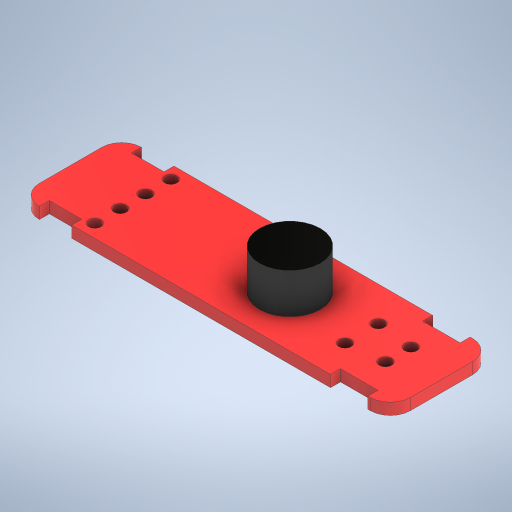
# Autodesk Inventor part: femtobuck-sparkfun
Saved by Autodesk Inventor 2023 (Build 270158030, 158C)
## iProperties
Created: 2023-08-09
Part Number: femtobuck-sparkfun
Material: Generic
Document SubType Name: Modeling
Designer: Imogen Heard
Density: 1 g/cm^3
Appearance: Default
Author: Imogen Heard
Autodesk Inventor part; units mm, degrees
ref_plane "YZ Plane" through (0, 0, 0) normal (1, 0, 0) x (0, 1, 0)
ref_plane "XZ Plane" through (0, 0, 0) normal (0, 1, 0) x (-1, 0, 0)
ref_plane "XY Plane" through (0, 0, 0) normal (0, 0, 1) x (1, 0, 0)
sketch "Sketch1" plane through (0, 0, 0) normal (0, 1, 0) x (-1, 0, 0)
  line L0 (-37.2, -2) -> (-37.2, -8.25)
  line L1 (0, -8.25) -> (0, -2)
  circle A0 centre (-6.25, -8.935) radius 0.625
  circle A1 centre (-6.25, -6.395) radius 0.625
  circle A2 centre (-6.25, -3.855) radius 0.625
  circle A3 centre (-6.25, -1.315) radius 0.625
  circle A4 centre (-32.85, -6.4) radius 0.625
  circle A5 centre (-32.85, -3.855) radius 0.625
  circle A6 centre (-29.2, -6.8) radius 0.625
  circle A7 centre (-29.2, -3.45) radius 0.625
  arc A8 (-2, -10.25) -> (0, -8.25) centre (-2, -8.25) ccw
  arc A9 (0, -2) -> (-2, 0) centre (-2, -2) ccw
  arc A10 (-35.2, 0) -> (-37.2, -2) centre (-35.2, -2) ccw
  arc A11 (-37.2, -8.25) -> (-35.2, -10.25) centre (-35.2, -8.25) ccw
  line L2 (-34.95, -10.25) -> (-34.95, -9.25)
  line L3 (-34.95, -9.25) -> (-31.2, -9.25)
  line L4 (-31.2, -9.25) -> (-31.2, -10.25)
  line L5 (-34.95, 0) -> (-34.95, -1)
  line L6 (-34.95, -1) -> (-31.2, -1)
  line L7 (-31.2, -1) -> (-31.2, 0)
  line L8 (-5.25, -10.25) -> (-5.25, -9.25)
  line L9 (-5.25, -9.25) -> (-2, -9.25)
  line L10 (-2, -9.25) -> (-2, -10.25)
  line L11 (-5.25, 0) -> (-5.25, -1)
  line L12 (-5.25, -1) -> (-2, -1)
  line L13 (-2, -1) -> (-2, 0)
  line L14 (-5.25, 0) -> (-31.2, 0)
  line L15 (-34.95, 0) -> (-35.2, 0)
  line L16 (-35.2, -10.25) -> (-34.95, -10.25)
  line L17 (-31.2, -10.25) -> (-5.25, -10.25)
  point P0 (0, 0)
  point P1 (0, 0)
  point P2 (-37.2, -10.25)
  point P3 (-37.2, -0.005)
  point P4 (-37.2, -5.125)
  point P5 (-33.075, -1)
  dimension "d0" = 37.2
  dimension "d2" = 4.35
  dimension "d3" = 8
  dimension "d4" = 3.85
  dimension "d5" = 3.85
  dimension "d6" = 2.545
  dimension "d7" = 2.54
  dimension "d8" = 2.54
  dimension "d9" = 2.54
  dimension "d10" = 2
  dimension "d11" = 6.25
  dimension "d14" = 1.25
  dimension "d17" = 2.25
  dimension "d18" = 6
  dimension "d22" = 5.25
  dimension "d23" = 2
  dimension "d24" = 10.25
  dimension "d25" = 1
  dimension "d26" = 3.75
  dimension "d27" = 1
  dimension "d28" = 2
  dimension "d29" = 2
  dimension "d30" = 1.315
  dimension "d31" = 1.315
  dimension "d32" = 3.45
  dimension "d33" = 3.45
  dimension "d34" = 3.85
  dimension "d35" = 1.25
  dimension "d36" = 3.855
  constraints: 36 end point, 12 centre point, 12 tangent, 10 equal radius, 9 parallel, 9 vertical alignment, 8 point on circle, 5 point on line, 2 coincident, 2 horizontal, 2 horizontal alignment, 2 midpoint, 2 perpendicular
  measures "d0" distance between parallel lines of L0 L1
  measures "d2" horizontal distance of A4.centre point (-37.2, -5.125)
  measures "d3" distance from line of A6.centre L0
  measures "d4" vertical distance of point (-37.2, -10.25) A4.centre
  measures "d5" vertical distance of point (-37.2, -0.005) A5.centre
  measures "d6" distance of A5.centre A4.centre
  measures "d7" distance of A1.centre A0.centre
  measures "d8" distance of A2.centre A1.centre
  measures "d9" distance of A3.centre A2.centre
  measures "d10" radius of A8
  measures "d11" distance from line of L1 A0.centre
  measures "d14" diameter of A0
  measures "d17" distance between parallel lines of L2 L0
  measures "d18" distance between parallel lines of L0 L4
  measures "d22" distance between parallel lines of L8 L1
  measures "d23" distance between parallel lines of L1 L10
  measures "d24" distance between parallel lines of L14 L17
  measures "d25" distance between parallel lines of L17 L3
  measures "d26" distance of L5.end L6.end
  measures "d27" distance between parallel lines of L14 L12
  measures "d28" horizontal distance of point (0, 0) A9.centre
  measures "d29" horizontal distance of point (0, 0) A9.centre
  measures "d30" distance from line of L17 A0.centre
  measures "d31" distance from line of L14 A3.centre
  measures "d32" distance from line of L14 A7.centre
  measures "d33" distance from line of L17 A6.centre
  measures "d34" distance from line of L17 A4.centre
  measures "d35" diameter of A5
  measures "d36" distance from line of L14 A5.centre
extrude "Extrusion1" add sketch "Sketch1" along normal blind 1.15
sketch "Sketch2" plane through (0, 1.15, 0) normal (0, 1, 0) x (1, 0, 0)
  circle A0 centre (22, 5.125) radius 3.05
  line L0 (37.2, 2) -> (37.2, 8.25) projected
  line L1 (5.25, 0) -> (31.2, 0) projected
  line L2 (31.2, 10.25) -> (5.25, 10.25) projected
  point P0 (0, 0)
  dimension "d39" = 6.1
  dimension "d40" = 15.2
  dimension "d41" = 5.125
  dimension "d42" = 5.125
  constraints: 1 centre point
  measures "d39" diameter of A0
  measures "d40" distance from line of L0 A0.centre
  measures "d41" distance from line of L1 A0.centre
  measures "d42" distance from line of L2 A0.centre
extrude "Extrusion2" add sketch "Sketch2" along normal blind 4
equation "\"d5\" = d4"
equation "\"d8\" = d7"
equation "\"d9\" = d7"
equation "\"d13\" = d12"
equation "\"d20\" = d19"
equation "\"d12\" = 3.45"
equation "\"d19\" = 1"
body "Solid1"
